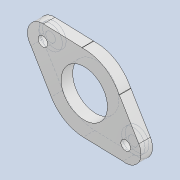
# Autodesk Inventor part: モータマウント2
Saved by Autodesk Inventor 2020 (Build 240168000, 168)
## iProperties
Created: 2020-11-01
Part Number: モータマウント2
Material: アルミニウム 2014-T4
Document SubType Name: Modeling
Designer: AA19065
Density: 2.8 g/cm^3
Appearance: サテン
Author: AA19065
Autodesk Inventor part; units mm, degrees
ref_plane "YZ Plane" through (0, 0, 0) normal (1, 0, 0) x (0, 1, 0)
ref_plane "XZ Plane" through (0, 0, 0) normal (0, 1, 0) x (-1, 0, 0)
ref_plane "XY Plane" through (0, 0, 0) normal (0, 0, 1) x (1, 0, 0)
sketch "スケッチ1" plane through (0, 0, 0) normal (0, 0, 1) x (1, 0, 0)
  line L0 (0, 0) -> (-26.8716, 23) construction
  line L1 (32.7705, -12.2921) -> (0, 0) construction
  circle A0 centre (0, 0) radius 8
  circle A1 centre (0, 0) radius 6.025
  circle A2 centre (0, 0) radius 10
  line L2 (30.3398, -14.0505) -> (4.0407, -9.1473)
  line L3 (9.0597, 4.2333) -> (32.0958, -9.369)
  line L4 (-23.9861, 23.821) -> (-0.5538, 9.9847)
  line L5 (-9.9505, -0.9938) -> (-27.2374, 20.0224)
  circle A3 centre (-10.7763, 6.3341) radius 3.05
  circle A4 centre (-10.7763, 6.3341) radius 1.25
  circle A5 centre (10.7763, -6.3341) radius 3.05
  circle A6 centre (10.7763, -6.3341) radius 1.25
  arc A7 (-10.6465, 10.3494) -> (-13.8789, 3.7821) centre (-10.7763, 6.3341) ccw
  arc A8 (10.0432, -10.2664) -> (14.2097, -4.2819) centre (10.7763, -6.3341) ccw
  line L6 (-10.6465, 10.3494) -> (0.3231, 9.9948)
  line L7 (8.5835, 5.1307) -> (14.2097, -4.2819)
  line L8 (10.0432, -10.2664) -> (-0.2617, -9.9966)
  line L9 (-8.5971, -5.1078) -> (-13.8789, 3.7821)
  point P0 (-0.6227, 10.0254)
  point P1 (9.1526, 4.1785)
  dimension "d0" = 12.05
  dimension "d5" = 2.5
  constraints: 20 end point, 8 centre point, 4 point on circle, 4 tangent, 2 coincident, 2 point on line, 1 equal radius, 30 other
  measures "d0" diameter of A1
  measures "d5" diameter of A4
extrude "押し出し1" add sketch "スケッチ1" along normal blind 3 contours A0 | A2 A5 A3 | A2 L3 L7 A8 L2 A5 | A5 A2 | A2 A5 | L2 L8 A2 | A2 A3 L5 A7 L6 L4 | A3 A2 | A2 A3 | L9 L5 A2
extrude "押し出し2" cut sketch "スケッチ1" along normal blind 1 contours A5 A2 | A2 A5 | A3 A2 | A2 A3 | A4 | A6
